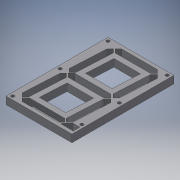
# Autodesk Inventor part: Segment_V4
Saved by Autodesk Inventor 2016 SP2 (Build 200236200, 236)
## iProperties
Created: 2018-06-10
Part Number: Segment_V4
Material: Generisch
Document SubType Name: Modeling
Designer: Nils
Density: 1 g/cm^3
Appearance: Vorgabe
Author: Nils
Autodesk Inventor part; units mm, degrees
ref_plane "YZ Plane" through (0, 0, 0) normal (1, 0, 0) x (0, 1, 0)
ref_plane "XZ Plane" through (0, 0, 0) normal (0, 1, 0) x (-1, 0, 0)
ref_plane "XY Plane" through (0, 0, 0) normal (0, 0, 1) x (1, 0, 0)
sketch "Skizze1" plane through (0, 0, 0) normal (0, 0, 1) x (1, 0, 0)
  line L0 (0, 0) -> (99.0002, 0)
  line L1 (99.0002, 0) -> (99.0002, 153.201)
  line L2 (99.0002, 153.201) -> (0, 153.201)
  line L3 (0, 153.201) -> (0, 0)
  line L4 (14.1667, 10) -> (19.1667, 5)
  line L5 (19.1667, 5) -> (73.1667, 5)
  line L6 (73.1667, 5) -> (78.1667, 10)
  line L7 (78.1667, 10) -> (73.1667, 15)
  line L8 (19.1667, 15) -> (14.1667, 10)
  line L9 (13, 11.1667) -> (18, 16.1667)
  line L10 (13, 11.1667) -> (8, 16.1667)
  line L11 (20.8261, 70.0927) -> (15.8261, 75.0927)
  line L12 (15.8261, 75.0927) -> (10.8261, 70.0927)
  line L13 (10.8261, 70.0927) -> (8, 16.1667)
  line L14 (19.1667, 15) -> (20.1667, 15)
  line L15 (20.1667, 15) -> (20.1667, 15.2)
  line L16 (20.1667, 15.2) -> (72.1667, 15.2)
  line L17 (72.1667, 15.2) -> (72.1667, 15)
  line L18 (72.1667, 15) -> (73.1667, 15)
  line L19 (18, 16.1667) -> (18.0523, 17.1654)
  line L20 (18.0523, 17.1654) -> (18.2521, 17.1549)
  line L21 (18.2521, 17.1549) -> (20.9735, 69.0836)
  line L22 (20.9735, 69.0836) -> (20.7738, 69.0941)
  line L23 (20.7738, 69.0941) -> (20.8261, 70.0927)
  line L24 (77.5002, 5) -> (77.5002, 7)
  line L25 (77.5002, 7) -> (85.5002, 15)
  line L26 (85.5002, 15) -> (96.0002, 15)
  line L27 (96.0002, 15) -> (96.0002, 5)
  line L28 (96.0002, 5) -> (77.5002, 5)
  line L29 (74.3335, 16.1667) -> (79.3335, 11.1667)
  line L30 (79.3335, 11.1667) -> (84.3335, 16.1667)
  line L31 (84.3335, 16.1667) -> (87.1596, 70.0927)
  line L32 (87.1596, 70.0927) -> (82.1596, 75.0927)
  line L33 (82.1596, 75.0927) -> (77.1596, 70.0927)
  line L34 (77.1596, 70.0927) -> (77.1073, 69.0941)
  line L35 (77.1073, 69.0941) -> (76.9075, 69.1046)
  line L36 (76.9075, 69.1046) -> (74.1861, 17.1758)
  line L37 (74.1861, 17.1758) -> (74.3858, 17.1654)
  line L38 (74.3858, 17.1654) -> (74.3335, 16.1667)
  line L39 (16.9929, 76.2594) -> (21.9929, 71.2594)
  line L40 (21.9929, 71.2594) -> (22.9929, 71.2594)
  line L41 (22.9929, 71.2594) -> (22.9929, 71.0594)
  line L42 (22.9929, 71.0594) -> (74.9929, 71.0594)
  line L43 (74.9929, 71.0594) -> (74.9929, 71.2594)
  line L44 (74.9929, 71.2594) -> (75.9929, 71.2594)
  line L45 (75.9929, 71.2594) -> (80.9929, 76.2594)
  line L46 (80.9929, 76.2594) -> (75.9929, 81.2594)
  line L47 (75.9929, 81.2594) -> (21.9929, 81.2594)
  line L48 (21.9929, 81.2594) -> (16.9929, 76.2594)
  line L49 (16.5083, 78.1083) -> (21.5083, 83.1083)
  line L50 (21.5083, 83.1083) -> (21.5606, 84.1069)
  line L51 (21.5606, 84.1069) -> (21.7603, 84.0965)
  line L52 (21.7603, 84.0965) -> (24.4818, 136.0252)
  line L53 (24.4818, 136.0252) -> (24.2821, 136.0357)
  line L54 (24.2821, 136.0357) -> (24.3344, 137.0343)
  line L55 (24.3344, 137.0343) -> (19.3344, 142.0343)
  line L56 (19.3344, 142.0343) -> (14.3344, 137.0343)
  line L57 (14.3344, 137.0343) -> (11.5083, 83.1083)
  line L58 (11.5083, 83.1083) -> (16.5083, 78.1083)
  line L59 (77.8417, 83.1083) -> (82.8417, 78.1083)
  line L60 (82.8417, 78.1083) -> (87.8417, 83.1083)
  line L61 (87.8417, 83.1083) -> (90.6679, 137.0343)
  line L62 (90.6679, 137.0343) -> (85.6679, 142.0343)
  line L63 (85.6679, 142.0343) -> (80.6679, 137.0343)
  line L64 (80.6679, 137.0343) -> (80.6155, 136.0357)
  line L65 (80.6155, 136.0357) -> (80.4158, 136.0461)
  line L66 (80.4158, 136.0461) -> (77.6943, 84.1174)
  line L67 (77.6943, 84.1174) -> (77.894, 84.1069)
  line L68 (77.894, 84.1069) -> (77.8417, 83.1083)
  line L69 (25.5011, 148.201) -> (20.5011, 143.201)
  line L70 (20.5011, 143.201) -> (25.5011, 138.201)
  line L71 (25.5011, 138.201) -> (26.5011, 138.201)
  line L72 (26.5011, 138.201) -> (26.5011, 138.001)
  line L73 (26.5011, 138.001) -> (78.5011, 138.001)
  line L74 (78.5011, 138.001) -> (78.5011, 138.201)
  line L75 (78.5011, 138.201) -> (79.5011, 138.201)
  line L76 (79.5011, 138.201) -> (84.5011, 143.201)
  line L77 (84.5011, 143.201) -> (79.5011, 148.201)
  line L78 (79.5011, 148.201) -> (25.5011, 148.201)
  line L79 (68.5797, 63.0594) -> (28.6688, 63.0594)
  line L80 (28.6688, 63.0594) -> (26.5799, 23.2)
  line L81 (26.5799, 23.2) -> (66.4908, 23.2)
  line L82 (66.4908, 23.2) -> (68.5797, 63.0594)
  line L83 (72.088, 130.001) -> (69.9528, 89.2594)
  line L84 (69.9528, 89.2594) -> (30.0419, 89.2594)
  line L85 (30.0419, 89.2594) -> (32.1771, 130.001)
  line L86 (32.1771, 130.001) -> (72.088, 130.001)
  dimension "d1" = 10
  dimension "d3" = 135
  dimension "d6" = 5
  dimension "d9" = 3
  dimension "d10" = 8
  dimension "d37" = 52
  dimension "d39" = 1
  dimension "d40" = 0.2
  dimension "d59" = 0
  dimension "d66" = 0
  dimension "d68" = 5
  dimension "d70" = 1.65
  dimension "d71" = 1.65
  dimension "d74" = 0
  dimension "d76" = 0
  dimension "d80" = 0
  dimension "d81" = 0
  dimension "d82" = 1.65
  dimension "d84" = 1.65
  dimension "d85" = 1.65
  dimension "d87" = 10
  dimension "d88" = 2
  dimension "d89" = 1.65
  dimension "d90" = 0
  dimension "d91" = 18.5
  dimension "d92" = 3
  dimension "d168" = 8
  dimension "d169" = 8
  dimension "d170" = 8
  dimension "d171" = 8
  dimension "d172" = 8
  dimension "d173" = 8
  dimension "d174" = 8
  dimension "d175" = 8
  constraints: 174 end point, 54 equal length, 47 parallel, 19 perpendicular, 8 horizontal, 6 collinear, 5 vertical, 3 point on line
  measures "d1" distance from line of L5 L8.start
  measures "d3" angle of L5 L4
  measures "d6" distance between parallel lines of L0 L5
  measures "d9" angle of L13 L3
  measures "d10" distance from line of L3 L10.end
  measures "d37" distance of L15.end L16.end
  measures "d39" distance of L8.start L14.end
  measures "d40" distance of L14.end L15.end
  measures "d59" distance between parallel lines of L30 L6
  measures "d66" distance between parallel lines of L31 L61
  measures "d68" distance between parallel lines of L2 L78
  measures "d70" distance between parallel lines of L8 L9
  measures "d71" distance between parallel lines of L29 L7
  measures "d74" distance between parallel lines of L48 L12
  measures "d76" distance between parallel lines of L13 L57
  measures "d80" distance between parallel lines of L56 L69
  measures "d81" distance between parallel lines of L77 L62
  measures "d82" distance between parallel lines of L70 L55
  measures "d84" distance between parallel lines of L39 L11
  measures "d85" distance between parallel lines of L48 L49
  measures "d87" distance between parallel lines of L28 L26
  measures "d88" distance of L24.start L24.end
  measures "d89" distance between parallel lines of L25 L30
  measures "d90" distance between parallel lines of L5 L28
  measures "d91" distance of L27.end L24.start
  measures "d92" distance between parallel lines of L1 L27
  measures "d168" distance between parallel lines of L21 L80
  measures "d169" distance between parallel lines of L82 L36
  measures "d170" distance between parallel lines of L16 L81
  measures "d171" distance between parallel lines of L42 L79
  measures "d172" distance between parallel lines of L47 L84
  measures "d173" distance between parallel lines of L66 L83
  measures "d174" distance between parallel lines of L73 L86
  measures "d175" distance between parallel lines of L52 L85
extrude "Extrusion1" add sketch "Skizze1" along normal blind 10.5
chamfer "Fase3" distance 10.5 angle 10 1 edges at (46.1667, 15.2, 0) measured on face at (46.1667, 15.2, 0.5)
chamfer "Fase4" distance 10.5 angle 10 1 edges at (19.6128, 43.1193, 0) measured on face at (19.6128, 43.1193, 0.5)
chamfer "Fase5" distance 10.5 angle 10 1 edges at (75.5468, 43.1402, 0) measured on face at (75.5468, 43.1402, 0.5)
chamfer "Fase6" distance 10.5 angle 10 1 edges at (48.9929, 71.0594, 0) measured on face at (48.9929, 71.0594, 0.5)
chamfer "Fase7" distance 10.5 angle 10 1 edges at (79.0551, 110.0818, 0) measured on face at (79.0551, 110.0818, 0.5)
chamfer "Fase8" distance 10.5 angle 10 1 edges at (23.1211, 110.0608, 0) measured on face at (23.1211, 110.0608, 0.5)
chamfer "Fase9" distance 10.5 angle 10 1 edges at (52.5011, 138.001, 0) measured on face at (52.5011, 138.001, 0.5)
chamfer "Fase10" distance 10.5 angle 10 1 edges at (86.7502, 5, 0) measured on face at (86.7502, 5, 0.5)
sketch "Skizze2" plane through (0, 0, 0) normal (0, 0, -1) x (-1, 0, 0)
  line L0 (0, 0) -> (-99.0002, 0) projected
  line L1 (0, 153.201) -> (0, 0) projected
  circle A0 centre (-21.8667, 15.3514) radius 1.75
  circle A1 centre (-18.4923, 18.8446) radius 1.75
  circle A2 centre (-70.4667, 15.3514) radius 1.75
  circle A3 centre (-21.0358, 67.378) radius 1.75
  line L2 (-20.1667, 17.0514) -> (-72.1667, 17.0514) construction
  line L3 (-20.1667, 17.0514) -> (-20.1667, 15) projected
  line L4 (-72.1667, 17.0514) -> (-72.1667, 15) projected
  line L5 (-20.101, 17.058) -> (-18.0523, 17.1654) projected
  line L6 (-22.8224, 68.9867) -> (-20.7738, 69.0941) projected
  line L7 (-96.0002, 3.1486) -> (-96.0002, 15) construction
  line L8 (-96.0002, 15) -> (-85.5002, 15) construction
  line L9 (-85.5002, 15) -> (-77.5002, 7) construction
  line L10 (-77.5002, 3.1486) -> (-77.5002, 7) construction
  line L11 (-96.0002, 3.1486) -> (-77.5002, 3.1486) construction
  line L12 (-78.5011, 136.1496) -> (-78.5011, 138.201) projected
  line L13 (-78.5011, 138.201) -> (-79.5011, 138.201) projected
  line L14 (-79.5011, 138.201) -> (-84.5011, 143.201) projected
  line L15 (-84.5011, 143.201) -> (-79.5011, 148.201) projected
  line L16 (-79.5011, 148.201) -> (-25.5011, 148.201) projected
  line L17 (-25.5011, 148.201) -> (-20.5011, 143.201) projected
  line L18 (-20.5011, 143.201) -> (-25.5011, 138.201) projected
  line L19 (-25.5011, 138.201) -> (-26.5011, 138.201) projected
  line L20 (-26.5011, 136.1496) -> (-26.5011, 138.201) projected
  line L21 (-78.5011, 136.1496) -> (-26.5011, 136.1496) construction
  line L22 (-26.3307, 135.9283) -> (-24.2821, 136.0357) projected
  line L23 (-24.2821, 136.0357) -> (-24.3344, 137.0343) projected
  line L24 (-24.3344, 137.0343) -> (-19.3344, 142.0343) projected
  line L25 (-19.3344, 142.0343) -> (-14.3344, 137.0343) projected
  line L26 (-14.3344, 137.0343) -> (-11.5083, 83.1083) construction
  line L27 (-11.5083, 83.1083) -> (-16.5083, 78.1083) projected
  line L28 (-16.5083, 78.1083) -> (-21.5083, 83.1083) projected
  line L29 (-21.5083, 83.1083) -> (-21.5606, 84.1069) projected
  line L30 (-23.6092, 83.9996) -> (-21.5606, 84.1069) projected
  line L31 (-26.3307, 135.9283) -> (-23.6092, 83.9996) projected
  line L32 (-75.8454, 84.2143) -> (-77.894, 84.1069) projected
  line L33 (-77.894, 84.1069) -> (-77.8417, 83.1083) projected
  line L34 (-77.8417, 83.1083) -> (-82.8417, 78.1083) construction
  line L35 (-82.8417, 78.1083) -> (-87.8417, 83.1083) construction
  line L36 (-87.8417, 83.1083) -> (-90.6679, 137.0343) construction
  line L37 (-90.6679, 137.0343) -> (-85.6679, 142.0343) projected
  line L38 (-85.6679, 142.0343) -> (-80.6679, 137.0343) projected
  line L39 (-80.6679, 137.0343) -> (-80.6155, 136.0357) projected
  line L40 (-78.5669, 136.143) -> (-80.6155, 136.0357) projected
  line L41 (-75.8454, 84.2143) -> (-78.5669, 136.143) construction
  line L42 (-74.9929, 69.208) -> (-74.9929, 71.2594) projected
  line L43 (-74.9929, 71.2594) -> (-75.9929, 71.2594) projected
  line L44 (-75.9929, 71.2594) -> (-80.9929, 76.2594) construction
  line L45 (-80.9929, 76.2594) -> (-75.9929, 81.2594) construction
  line L46 (-75.9929, 81.2594) -> (-21.9929, 81.2594) construction
  line L47 (-21.9929, 81.2594) -> (-16.9929, 76.2594) projected
  line L48 (-16.9929, 76.2594) -> (-21.9929, 71.2594) projected
  line L49 (-21.9929, 71.2594) -> (-22.9929, 71.2594) projected
  line L50 (-22.9929, 69.208) -> (-22.9929, 71.2594) projected
  line L51 (-74.9929, 69.208) -> (-22.9929, 69.208) construction
  line L52 (-72.3372, 17.2727) -> (-74.3858, 17.1654) projected
  line L53 (-74.3858, 17.1654) -> (-74.3335, 16.1667) projected
  line L54 (-74.3335, 16.1667) -> (-79.3335, 11.1667) projected
  line L55 (-79.3335, 11.1667) -> (-84.3335, 16.1667) projected
  line L56 (-84.3335, 16.1667) -> (-87.1596, 70.0927) construction
  line L57 (-87.1596, 70.0927) -> (-82.1596, 75.0927) construction
  line L58 (-82.1596, 75.0927) -> (-77.1596, 70.0927) construction
  line L59 (-77.1596, 70.0927) -> (-77.1073, 69.0941) projected
  line L60 (-75.0586, 69.2015) -> (-77.1073, 69.0941) projected
  line L61 (-72.3372, 17.2727) -> (-75.0586, 69.2015) construction
  line L62 (-22.8224, 68.9867) -> (-20.7738, 69.0941) projected
  line L63 (-20.7738, 69.0941) -> (-20.8261, 70.0927) projected
  line L64 (-20.8261, 70.0927) -> (-15.8261, 75.0927) projected
  line L65 (-15.8261, 75.0927) -> (-10.8261, 70.0927) projected
  line L66 (-10.8261, 70.0927) -> (-8, 16.1667) construction
  line L67 (-8, 16.1667) -> (-13, 11.1667) projected
  line L68 (-13, 11.1667) -> (-18, 16.1667) projected
  line L69 (-18, 16.1667) -> (-18.0523, 17.1654) projected
  line L70 (-20.101, 17.058) -> (-18.0523, 17.1654) projected
  line L71 (-22.8224, 68.9867) -> (-20.101, 17.058) construction
  line L72 (-20.1667, 17.0514) -> (-20.1667, 15) projected
  line L73 (-20.1667, 15) -> (-19.1667, 15) projected
  line L74 (-19.1667, 15) -> (-14.1667, 10) projected
  line L75 (-14.1667, 10) -> (-19.1667, 5) projected
  line L76 (-19.1667, 5) -> (-73.1667, 5) construction
  line L77 (-73.1667, 5) -> (-78.1667, 10) projected
  line L78 (-78.1667, 10) -> (-73.1667, 15) projected
  line L79 (-73.1667, 15) -> (-72.1667, 15) projected
  line L80 (-72.1667, 17.0514) -> (-72.1667, 15) projected
  line L81 (-20.1667, 17.0514) -> (-72.1667, 17.0514) construction
  line L82 (0, 0) -> (-99.0002, 0) projected
  line L83 (0, 153.201) -> (0, 0) projected
  line L84 (-99.0002, 153.201) -> (0, 153.201) projected
  line L85 (-99.0002, 0) -> (-99.0002, 153.201) projected
  circle A4 centre (-74.1238, 18.8814) radius 1.75
  circle A5 centre (-76.6673, 67.4148) radius 1.75
  circle A6 centre (-73.2929, 70.908) radius 1.75
  circle A7 centre (-24.6929, 70.908) radius 1.75
  circle A8 centre (-77.6321, 85.823) radius 1.75
  circle A9 centre (-80.1756, 134.3564) radius 1.75
  circle A10 centre (-76.8011, 137.8496) radius 1.75
  circle A11 centre (-28.2011, 137.8496) radius 1.75
  circle A12 centre (-24.544, 134.3196) radius 1.75
  circle A13 centre (-22.0005, 85.7862) radius 1.75
  circle A14 centre (-79.2002, 4.8486) radius 1.75
  circle A15 centre (-94.3002, 4.8486) radius 1.75
  line L86 (-26.5799, 23.2) -> (-66.4908, 23.2) projected
  line L87 (-66.4908, 23.2) -> (-68.5797, 63.0594) projected
  line L88 (-68.5797, 63.0594) -> (-28.6688, 63.0594) projected
  line L89 (-28.6688, 63.0594) -> (-26.5799, 23.2) projected
  line L90 (-30.0419, 89.2594) -> (-69.9528, 89.2594) projected
  line L91 (-69.9528, 89.2594) -> (-72.088, 130.001) projected
  line L92 (-72.088, 130.001) -> (-32.1771, 130.001) projected
  line L93 (-32.1771, 130.001) -> (-30.0419, 89.2594) projected
  dimension "d23" = 3.5
  dimension "d24" = 3.5
  dimension "d25" = 3.5
  dimension "d26" = 3.5
  dimension "d48" = 1.7
  dimension "d49" = 1.7
  dimension "d50" = 1.7
  dimension "d51" = 1.7
  dimension "d53" = 1.7
  dimension "d55" = 1.7
  dimension "d111" = 3.5
  dimension "d112" = 3.5
  dimension "d113" = 3.5
  dimension "d114" = 3.5
  dimension "d115" = 3.5
  dimension "d116" = 3.5
  dimension "d117" = 3.5
  dimension "d118" = 3.5
  dimension "d119" = 3.5
  dimension "d120" = 3.5
  dimension "d121" = 3.5
  dimension "d122" = 3.5
  dimension "d123" = 1.7
  dimension "d124" = 1.7
  dimension "d125" = 1.7
  dimension "d126" = 1.7
  dimension "d127" = 1.7
  dimension "d128" = 1.7
  dimension "d129" = 1.7
  dimension "d130" = 1.7
  dimension "d131" = 1.7
  dimension "d132" = 1.7
  dimension "d133" = 1.7
  dimension "d134" = 1.7
  dimension "d135" = 1.7
  dimension "d136" = 1.7
  dimension "d137" = 1.7
  dimension "d138" = 1.7
  dimension "d139" = 1.7
  dimension "d140" = 1.7
  dimension "d141" = 1.7
  dimension "d142" = 1.7
  dimension "d143" = 1.7
  dimension "d144" = 1.7
  dimension "d145" = 1.7
  dimension "d146" = 1.7
  constraints: 16 centre point
  measures "d23" diameter of A0
  measures "d24" diameter of A1
  measures "d25" diameter of A2
  measures "d26" diameter of A3
  measures "d48" distance from line of L2 A0.centre
  measures "d49" distance from line of L3 A0.centre
  measures "d50" distance from line of L2 A2.centre
  measures "d51" distance from line of L4 A2.centre
  measures "d53" distance from line of L5 A1.centre
  measures "d55" distance from line of L6 A3.centre
  measures "d111" diameter of A14
  measures "d112" diameter of A15
  measures "d113" diameter of A4
  measures "d114" diameter of A5
  measures "d115" diameter of A6
  measures "d116" diameter of A7
  measures "d117" diameter of A8
  measures "d118" diameter of A13
  measures "d119" diameter of A9
  measures "d120" diameter of A10
  measures "d121" diameter of A11
  measures "d122" diameter of A12
  measures "d123" distance from line of A15.centre L7
  measures "d124" distance from line of L11 A15.centre
  measures "d125" distance from line of L11 A14.centre
  measures "d126" distance from line of L10 A14.centre
  measures "d127" distance from line of L61 A4.centre
  measures "d128" distance from line of L52 A4.centre
  measures "d129" distance from line of A5.centre L60
  measures "d130" distance from line of L61 A5.centre
  measures "d131" distance from line of L51 A6.centre
  measures "d132" distance from line of L42 A6.centre
  measures "d133" distance from line of L51 A7.centre
  measures "d134" distance from line of L50 A7.centre
  measures "d135" distance from line of L41 A8.centre
  measures "d136" distance from line of L32 A8.centre
  measures "d137" distance from line of L30 A13.centre
  measures "d138" distance from line of L31 A13.centre
  measures "d139" distance from line of L40 A9.centre
  measures "d140" distance from line of L41 A9.centre
  measures "d141" distance from line of L21 A10.centre
  measures "d142" distance from line of L12 A10.centre
  measures "d143" distance from line of L20 A11.centre
  measures "d144" distance from line of L21 A11.centre
  measures "d145" distance from line of L31 A12.centre
  measures "d146" distance from line of L22 A12.centre
extrude "Extrusion4" add sketch "Skizze2" along normal blind 0.8 contours L0 L85 L84 L1 | L22 A12 L31 | L30 L31 A13
sketch "Skizze3" plane through (0, 0, 10.5) normal (0, 0, 1) x (1, 0, 0)
  circle A0 centre (5, 5) radius 2.5
  circle A1 centre (5, 76.2594) radius 2.5
  circle A2 centre (94.0002, 76.2594) radius 2.5
  circle A3 centre (5, 148.201) radius 2.5
  circle A4 centre (94.0002, 148.201) radius 2.5
  line L0 (0, 153.201) -> (0, 0) projected
  line L1 (99.0002, 0) -> (0, 0) projected
  line L2 (99.0002, 153.201) -> (0, 153.201) projected
  line L3 (99.0002, 153.201) -> (99.0002, 0) projected
  circle A5 centre (94.0002, 20) radius 2.5
  line L4 (85.5002, 15) -> (96.0002, 15) projected
  point P0 (80.9929, 76.2594)
  point P1 (16.9929, 76.2594)
  dimension "d149" = 5
  dimension "d150" = 5
  dimension "d151" = 5
  dimension "d152" = 5
  dimension "d153" = 5
  dimension "d154" = 5
  dimension "d155" = 5
  dimension "d156" = 5
  dimension "d157" = 5
  dimension "d158" = 5
  dimension "d159" = 5
  dimension "d160" = 5
  dimension "d161" = 5
  dimension "d162" = 0
  dimension "d163" = 0
  dimension "d176" = 5
  dimension "d177" = 5
  dimension "d178" = 5
  constraints: 6 centre point
  measures "d149" diameter of A0
  measures "d150" diameter of A1
  measures "d151" diameter of A3
  measures "d152" diameter of A2
  measures "d153" diameter of A4
  measures "d154" distance from line of L0 A0.centre
  measures "d155" distance from line of L1 A0.centre
  measures "d156" distance from line of L0 A1.centre
  measures "d157" distance from line of L0 A3.centre
  measures "d158" distance from line of L2 A3.centre
  measures "d159" distance from line of L2 A4.centre
  measures "d160" distance from line of L3 A4.centre
  measures "d161" distance from line of L3 A2.centre
  measures "d162" vertical distance of point (80.993, 76.259) A2.centre
  measures "d163" vertical distance of point (16.993, 76.259) A1.centre
  measures "d176" diameter of A5
  measures "d177" distance from line of L3 A5.centre
  measures "d178" distance from line of L4 A5.centre
extrude "Extrusion5" cut sketch "Skizze3" against normal blind 3 contours A0 | A1 | A2 | A3 | A4 | A5
sketch "Skizze4" plane through (0, 0, -0.8) normal (0, 0, -1) x (-1, 0, 0)
  circle A0 centre (-94.0002, 76.2594) radius 2.5 projected
  circle A1 centre (-94.0002, 148.201) radius 2.5 projected
  circle A2 centre (-5, 148.201) radius 2.5 projected
  circle A3 centre (-5, 76.2594) radius 2.5 projected
  circle A4 centre (-5, 5) radius 2.5 projected
  circle A5 centre (-89.657, 25.2223) radius 2.5
  line L0 (-69.9528, 89.2594) -> (-72.088, 130.001) construction
  line L1 (-72.088, 130.001) -> (-32.1771, 130.001) construction
  line L2 (-32.1771, 130.001) -> (-30.0419, 89.2594) construction
  line L3 (-30.0419, 89.2594) -> (-69.9528, 89.2594) construction
  line L4 (-66.4908, 23.2) -> (-68.5797, 63.0594) construction
  line L5 (-68.5797, 63.0594) -> (-28.6688, 63.0594) construction
  line L6 (-28.6688, 63.0594) -> (-26.5799, 23.2) construction
  line L7 (-26.5799, 23.2) -> (-66.4908, 23.2) construction
  circle A6 centre (-94.3002, 4.8486) radius 1.75 construction
  circle A7 centre (-79.2002, 4.8486) radius 1.75 construction
  circle A8 centre (-22.0005, 85.7862) radius 1.75 construction
  circle A9 centre (-24.544, 134.3196) radius 1.75 construction
  circle A10 centre (-28.2011, 137.8496) radius 1.75 construction
  circle A11 centre (-80.1756, 134.3564) radius 1.75 construction
  circle A12 centre (-76.8011, 137.8496) radius 1.75 construction
  circle A13 centre (-77.6321, 85.823) radius 1.75 construction
  circle A14 centre (-24.6929, 70.908) radius 1.75 construction
  circle A15 centre (-76.6673, 67.4148) radius 1.75 construction
  circle A16 centre (-73.2929, 70.908) radius 1.75 construction
  circle A17 centre (-74.1238, 18.8814) radius 1.75 construction
  circle A18 centre (-21.0358, 67.378) radius 1.75 construction
  circle A19 centre (-70.4667, 15.3514) radius 1.75 construction
  circle A20 centre (-21.8667, 15.3514) radius 1.75 construction
  circle A21 centre (-18.4923, 18.8446) radius 1.75 construction
  line L8 (-99.0002, 0) -> (0, 0) construction
  line L9 (0, 0) -> (0, 153.201) construction
  line L10 (0, 153.201) -> (-99.0002, 153.201) construction
  line L11 (-99.0002, 153.201) -> (-99.0002, 0) construction
  line L12 (-99.0002, 28.9085) -> (-70.0916, 0) construction
  line L13 (-68.7779, 10) -> (-89.0002, 30.2223) construction
  line L14 (-89.0002, 30.2223) -> (-89.0002, 143.201) construction
  dimension "d179" = 5
  dimension "d180" = 5
  dimension "d183" = 8
  dimension "d184" = 4
  dimension "d185" = 5
  constraints: 1 centre point
  measures "d179" diameter of A0
  measures "d180" diameter of A5
  measures "d183" distance between parallel lines of L12 L13
  measures "d184" distance from line of A5.centre L12
  measures "d185" vertical distance of L13.end A5.centre
extrude "Extrusion6" cut sketch "Skizze4" against normal blind 3
equation "\"d71\" = d70"
equation "\"d82\" = d70"
equation "\"d84\" = d70"
equation "\"d85\" = d70"
equation "\"d89\" = d71"
equation "\"d24\" = d23"
equation "\"d25\" = d23"
equation "\"d26\" = d23"
equation "\"d49\" = d48"
equation "\"d50\" = d48"
equation "\"d51\" = d48"
equation "\"d53\" = d48"
equation "\"d55\" = d48"
equation "\"d111\" = d23"
equation "\"d112\" = d23"
equation "\"d113\" = d23"
equation "\"d114\" = d23"
equation "\"d115\" = d23"
equation "\"d116\" = d23"
equation "\"d117\" = d23"
equation "\"d118\" = d23"
equation "\"d119\" = d23"
equation "\"d120\" = d23"
equation "\"d121\" = d23"
equation "\"d122\" = d23"
equation "\"d123\" = d48"
equation "\"d124\" = d48"
